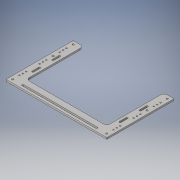
# Autodesk Inventor part: vrRig_v08p1_base
Saved by Autodesk Inventor 2016 (Build 200138000, 138)
## iProperties
Created: 2018-01-13
Part Number: vrRig_v08p1_base
Material: Generic
Document SubType Name: Modeling
Designer: harveylab
Density: 1 g/cm^3
Appearance: Default
Author: harveylab
Autodesk Inventor part; units mm, degrees
ref_plane "YZ Plane" through (0, 0, 0) normal (1, 0, 0) x (0, 1, 0)
ref_plane "XZ Plane" through (0, 0, 0) normal (0, 1, 0) x (-1, 0, 0)
ref_plane "XY Plane" through (0, 0, 0) normal (0, 0, 1) x (1, 0, 0)
sketch "Sketch1" plane through (0, 0, 0) normal (0, 1, 0) x (-1, 0, 0)
  circle A0 centre (368.3, 203.2) radius 2.54
  circle A1 centre (368.3, 241.3) radius 3.302
  circle A2 centre (368.3, 127) radius 2.54
  circle A3 centre (368.3, 88.9) radius 3.302
  circle A4 centre (368.3, 50.8) radius 2.54
  circle A5 centre (368.3, 12.7) radius 3.302
  line L0 (190.5, 244.602) -> (330.2, 244.602)
  line L1 (330.2, 244.602) -> (190.5, 244.602)
  arc A6 (330.2, 237.998) -> (330.2, 244.602) centre (330.2, 241.3) ccw
  line L2 (190.5, 237.998) -> (330.2, 237.998)
  line L3 (381, 251.46) -> (381, 2.54)
  line L4 (378.46, 0) -> (355.6, 0)
  line L5 (355.6, 0) -> (355.6, 0)
  circle A7 centre (368.3, 38.1) radius 2.54
  circle A8 centre (368.3, 63.5) radius 2.54
  circle A9 centre (368.3, 127) radius 2.54
  circle A10 centre (368.3, 114.3) radius 2.54
  circle A11 centre (368.3, 139.7) radius 2.54
  circle A12 centre (368.3, 203.2) radius 2.54
  circle A13 centre (368.3, 190.5) radius 2.54
  circle A14 centre (368.3, 215.9) radius 2.54
  line L6 (355.6, 0) -> (355.6, 25.4) construction
  line L7 (355.6, 25.4) -> (381, 25.4) construction
  line L8 (368.3, 88.9) -> (355.6, 88.9) construction
  arc A15 (352.298, 76.2) -> (358.902, 76.2) centre (355.6, 76.2) ccw
  arc A16 (358.902, 101.6) -> (352.298, 101.6) centre (355.6, 101.6) ccw
  line L9 (358.902, 76.2) -> (358.902, 101.6)
  line L10 (352.298, 101.6) -> (352.298, 76.2)
  line L11 (368.3, 139.7) -> (368.3, 165.1) construction
  line L12 (368.3, 165.1) -> (355.6, 165.1) construction
  arc A17 (352.298, 152.4) -> (358.902, 152.4) centre (355.6, 152.4) ccw
  arc A18 (358.902, 177.8) -> (352.298, 177.8) centre (355.6, 177.8) ccw
  line L13 (358.902, 152.4) -> (358.902, 177.8)
  line L14 (352.298, 177.8) -> (352.298, 152.4)
  arc A19 (342.9, 12.7) -> (355.6, 0) centre (355.6, 12.7) ccw
  line L15 (378.46, 254) -> (190.5, 254)
  arc A20 (378.46, 0) -> (381, 2.54) centre (378.46, 2.54) ccw
  arc A21 (381, 251.46) -> (378.46, 254) centre (378.46, 251.46) ccw
  line L16 (190.5, 228.6) -> (190.5, 159.7209) construction
  line L17 (330.2, 215.9) -> (190.5, 215.9)
  line L18 (342.9, 12.7) -> (342.9, 203.2)
  arc A22 (342.9, 203.2) -> (330.2, 215.9) centre (330.2, 203.2) ccw
  circle A23 centre (12.7, 203.2) radius 2.54
  circle A24 centre (12.7, 241.3) radius 3.302
  circle A25 centre (12.7, 127) radius 2.54
  circle A26 centre (12.7, 88.9) radius 3.302
  circle A27 centre (12.7, 50.8) radius 2.54
  circle A28 centre (12.7, 12.7) radius 3.302
  line L19 (190.5, 244.602) -> (50.8, 244.602)
  line L20 (50.8, 244.602) -> (190.5, 244.602)
  arc A29 (50.8, 244.602) -> (50.8, 237.998) centre (50.8, 241.3) ccw
  line L21 (190.5, 237.998) -> (50.8, 237.998)
  line L22 (0, 251.46) -> (0, 2.54)
  line L23 (2.54, 0) -> (25.4, 0)
  line L24 (25.4, 0) -> (25.4, 0)
  circle A30 centre (12.7, 38.1) radius 2.54
  circle A31 centre (12.7, 63.5) radius 2.54
  circle A32 centre (12.7, 139.7) radius 2.54
  circle A33 centre (12.7, 127) radius 2.54
  circle A34 centre (12.7, 114.3) radius 2.54
  circle A35 centre (12.7, 215.9) radius 2.54
  circle A36 centre (12.7, 203.2) radius 2.54
  circle A37 centre (12.7, 190.5) radius 2.54
  line L25 (25.4, 0) -> (25.4, 25.4) construction
  line L26 (25.4, 25.4) -> (0, 25.4) construction
  line L27 (12.7, 88.9) -> (25.4, 88.9) construction
  arc A38 (22.098, 76.2) -> (28.702, 76.2) centre (25.4, 76.2) ccw
  arc A39 (28.702, 101.6) -> (22.098, 101.6) centre (25.4, 101.6) ccw
  line L28 (22.098, 76.2) -> (22.098, 101.6)
  line L29 (28.702, 101.6) -> (28.702, 76.2)
  line L30 (12.7, 139.7) -> (12.7, 165.1) construction
  line L31 (12.7, 165.1) -> (25.4, 165.1) construction
  line L32 (22.098, 152.4) -> (22.098, 177.8)
  arc A40 (22.098, 152.4) -> (28.702, 152.4) centre (25.4, 152.4) ccw
  line L33 (28.702, 177.8) -> (28.702, 152.4)
  arc A41 (28.702, 177.8) -> (22.098, 177.8) centre (25.4, 177.8) ccw
  arc A42 (25.4, 0) -> (38.1, 12.7) centre (25.4, 12.7) ccw
  line L34 (2.54, 254) -> (190.5, 254)
  arc A43 (0, 2.54) -> (2.54, 0) centre (2.54, 2.54) ccw
  arc A44 (2.54, 254) -> (0, 251.46) centre (2.54, 251.46) ccw
  line L35 (50.8, 215.9) -> (190.5, 215.9)
  line L36 (38.1, 12.7) -> (38.1, 203.2)
  arc A45 (50.8, 215.9) -> (38.1, 203.2) centre (50.8, 203.2) ccw
  point P0 (381, 254)
  point P1 (381, 0)
  point P2 (342.9, 0)
  point P3 (342.9, 228.6)
  point P4 (0, 254)
  point P5 (0, 0)
  point P6 (38.1, 0)
  point P7 (38.1, 228.6)
  dimension "d2" = 12.7
  dimension "d3" = 228.6
  dimension "d6" = 25.4
  dimension "d7" = 25.4
  dimension "d8" = 12.7
  dimension "d10" = 25.4
  dimension "d12" = 12.7
  dimension "d17" = 12.7
  constraints: 74 end point, 52 symmetric about line, 46 centre point, 36 point on circle, 11 point on line, 11 tangent, 3 horizontal, 3 vertical, 2 perpendicular, 1 equal radius, 23 other
  measures "d2" distance of L4.end point (342.9, 0)
  measures "d3" distance of point (342.9, 0) point (342.9, 228.6)
  measures "d6" distance of L6.end L7.end
  measures "d7" distance of L6.start L6.end
  measures "d8" distance of L8.start L8.end
  measures "d10" distance of L11.start L11.end
  measures "d12" radius of A19
  measures "d17" radius of A22
extrude "Extrusion3" add sketch "Sketch1" along normal blind 6.35
body "Solid3"
